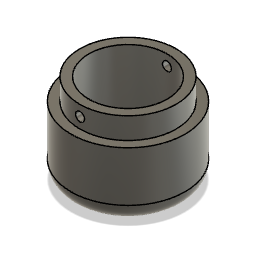
Projectile Housing (Autodesk Fusion 360 design; units mm, degrees)
Autodesk Fusion 360 part; units mm, degrees
sketch "Sketch1" plane through (0, 0, 0) normal (0, 0, 1) x (1, 0, 0) in component "Top Projectile"
  line L0 (13.7981, 10) -> (11.1635, 10)
  line L1 (22, 38) -> (32, 38)
  line L2 (32, 38) -> (32, 10)
  line L3 (32, 10) -> (22, 10)
  line L4 (22, 10) -> (22, 38)
  line L5 (27, 50) -> (22, 50)
  line L6 (22, 50) -> (22, 38)
  line L7 (22, 38) -> (27, 38)
  line L8 (27, 38) -> (27, 50)
  line L9 (0, 5.0221) -> (0, 0)
  line L10 (22, 10) -> (0, 10)
  line L11 (0, 10) -> (0, 0)
  line L12 (1.75, 0) -> (22.5, 0)
  line L13 (0, 0) -> (22, 0)
  arc A0 (22, 0) -> (32, 10) centre (22, 10) ccw
  circle A1 centre (0, 44) radius 2.5
  point P0 (32, 10)
  point P1 (22, 38)
  point P2 (27, 50)
  point P3 (0, 5.0221)
  dimension "d21" = 12
  dimension "d22" = 5
  dimension "d23" = 10
  dimension "d24" = 32
  dimension "d27" = 10
  dimension "d29" = 28
  dimension "d30" = 22
  dimension "d48" = 6
  dimension "d49" = 5
  dimension "d52" = 32
  constraint coincident L9.end L11.end
  constraint horizontal L0
  constraint horizontal L1
  constraint vertical L2
  constraint horizontal L3
  constraint vertical L4
  constraint coincident P0 L2.end
  constraint coincident P1 L1.start
  constraint horizontal L5
  constraint vertical L6
  constraint horizontal L7
  constraint vertical L8
  constraint coincident P2 L5.start
  constraint coincident P3 L9.start
  constraint parallel L4 L9
  constraint parallel L9 L11
  constraint parallel L10 L12
  constraint perpendicular L9 L13
  constraint tangent L13 A0
  measures "d21" distance of L1 P2
  measures "d22" distance of P2 L5.end
  measures "d23" distance of P1 L1.end
  measures "d24" horizontal distance of L9.end L2.end
  measures "d27" distance of L10.end L9.end
  measures "d29" distance of L1.end P0
  measures "d30" distance of L9.end L13.end
  measures "d48" distance of L5 A1.centre
  measures "d49" diameter of A1
  measures "d52" distance of L2 A1.centre
revolve "Revolve1" add sketch "Sketch1" angle 360 about axis through (0, 1.75, 0) along (0, 1, 0) contours L0 L3 L9 L10 L11 L12 L13 A0 | L1 L2 L3 L4 L7 | L1 L5 L6 L7 L8 makes body 1 in component "Top Projectile"
sketch "Sketch1 (2)" plane through (0, 0, 0) normal (0, 0, 1) x (1, 0, 0) in component "Bottom Projectile"
  line L0 (1.75, 0) -> (22.5, 0)
  line L1 (22, 38) -> (27, 38)
  line L2 (32, 10) -> (22, 10)
  line L3 (22, 10) -> (0, 10)
  line L4 (32, 38) -> (32, 10)
  arc A0 (22, 0) -> (32, 10) centre (22, 10) ccw
  line L5 (22, 10) -> (22, 38)
  line L6 (0, 5.0221) -> (0, 0)
  line L7 (13.7981, 10) -> (11.1635, 10)
  line L8 (22, 38) -> (32, 38)
  line L9 (0, 0) -> (22, 0)
  line L10 (0, 10) -> (0, 0)
  line L11 (27, 50) -> (32, 50)
  line L12 (32, 50) -> (32, 38)
  line L13 (32, 38) -> (27, 38)
  line L14 (27, 38) -> (27, 50)
  circle A1 centre (0, 44) radius 2.5
  line L15 (0, 1.75) -> (0, 22.5)
  point P0 (0, 5.0221)
  point P1 (22, 38)
  point P2 (32, 10)
  point P3 (27, 50)
  dimension "d41" = 10
  dimension "d42" = 32
  dimension "d43" = 10
  dimension "d44" = 28
  dimension "d45" = 22
  dimension "d46" = 5
  dimension "d47" = 12
  dimension "d56" = 5
  dimension "d57" = 32
  dimension "d58" = 6
  constraint coincident L6.end L9.start
  constraint horizontal L7
  constraint horizontal L8
  constraint vertical L4
  constraint horizontal L2
  constraint vertical L5
  constraint coincident P2 L2.start
  constraint coincident P1 L1.start
  constraint horizontal L1
  constraint coincident P0 L6.start
  constraint parallel L5 L6
  constraint parallel L6 L10
  constraint parallel L0 L3
  constraint perpendicular L6 L9
  constraint tangent A0 L9
  constraint horizontal L11
  constraint vertical L12
  constraint horizontal L13
  constraint vertical L14
  constraint coincident P3 L11.start
  constraint collinear L10 L15
  constraint collinear L0 L9
  measures "d41" distance of L4.start P1
  measures "d42" horizontal distance of L6.end P2
  measures "d43" distance of L3.end L6.end
  measures "d44" distance of L4.start P2
  measures "d45" distance of L6.end A0.start
  measures "d46" distance of L5 P3
  measures "d47" distance of L4.start L11.end
  measures "d56" diameter of A1
  measures "d57" distance of L12 A1.centre
  measures "d58" distance of L11 A1.centre
revolve "Revolve1'" add sketch "Sketch1 (2)" angle 360 about axis through (0, 1.75, 0) along (0, 1, 0) separate body contours L0 L2 L3 A0 L6 L7 L9 L10 L15 | L1 L2 L4 L5 L8 L13 | L8 L11 L12 L13 L14 makes body 2 in component "Bottom Projectile"
extrude "Extrude1" cut sketch "Sketch1" along normal through all and the other way through all contours A1 bodies 1 in component "Top Projectile"
extrude "Extrude1'" cut sketch "Sketch1" along normal through all and the other way through all contours A1 bodies 2 in component "Bottom Projectile"
component "Top Projectile" placed x (1, 0, 0) y (0, 1, 0) z (0, 0, 1) at (0, 0, 0)
component "Bottom Projectile" placed x (1, 0, 0) y (0, 1, 0) z (0, 0, 1) at (0, 0, 0)
equation "WallThickness = 10 mm" comment "Thickness of the projectile Wall"
equation "WallLength = 80 mm" comment "Length of the wall, not including the caps"
equation "d21 = WallLength * ( 3 / 10 ) * ( 1 / 2 )"
equation "d22 = WallThickness / 2"
equation "d23 = WallThickness"
equation "d24 = OutterRadius"
equation "OutterRadius = 32 mm"
equation "d27 = CapThickness"
equation "d29 = WallLength * ( 7 / 10 ) * ( 1 / 2 )"
equation "d30 = OutterRadius - WallThickness"
equation "CapThickness = 10 mm" comment "Thickness of the end caps"
equation "d41 = WallThickness"
equation "d42 = OutterRadius"
equation "d43 = CapThickness"
equation "d44 = WallLength * ( 7 / 10 ) * ( 1 / 2 )"
equation "d45 = OutterRadius - WallThickness"
equation "d46 = WallThickness / 2"
equation "d47 = WallLength * ( 3 / 10 ) * ( 1 / 2 )"
equation "d48 = WallLength * ( 3 / 10 ) * ( 1 / 4 )"
equation "d49 = InsertDiameter"
equation "InsertDiameter = 5 mm" comment "Diameter of the metal insert"
equation "d52 = OutterRadius"
equation "d56 = InsertDiameter"
equation "d57 = OutterRadius"
equation "d58 = WallLength * ( 3 / 10 ) * ( 1 / 4 )"
